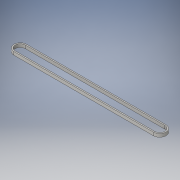
# Autodesk Inventor part: LiftLineWire
Saved by Autodesk Inventor 2016 (Build 200138000, 138)
## iProperties
Created: 2016-12-21
Part Number: LiftLineWire
Material: Generic
Document SubType Name: Modeling
Designer: RoboticsUser
Density: 1 g/cm^3
Appearance: Default
Author: RoboticsUser
Autodesk Inventor part; units mm, degrees
ref_plane "YZ Plane" through (0, 0, 0) normal (1, 0, 0) x (0, 1, 0)
ref_plane "XZ Plane" through (0, 0, 0) normal (0, 1, 0) x (-1, 0, 0)
ref_plane "XY Plane" through (0, 0, 0) normal (0, 0, 1) x (1, 0, 0)
sketch "Sketch1" plane through (0, 0, 0) normal (0, 1, 0) x (-1, 0, 0)
  line L0 (0, 0) -> (304.8083, 0)
  line L1 (304.8083, 0) -> (304.8083, -25.4)
  line L2 (304.8083, -25.4) -> (0, -25.4)
  line L3 (0, -25.4) -> (0, 0)
  dimension "d0" = 25.4
  constraints: 8 end point, 2 parallel, 1 horizontal, 1 perpendicular
  measures "d0" distance of L0.end L1.end
extrude "Extrusion1" add sketch "Sketch1" along normal blind 6.35
fillet "Fillet1" radius 12.7 1 edges at (-304.8083, 3.175, -25.4)
fillet "Fillet2" radius 12.7 1 edges at (-304.8083, 3.175, 0)
fillet "Fillet3" radius 12.7 1 edges at (0, 3.175, 0)
fillet "Fillet4" radius 12.7 1 edges at (0, 3.175, -25.4)
shell "Shell1" thickness 2.54 removed faces 2 at (-198.9723, 6.35, -8.4667) at (-198.9723, 0, -8.4667)
body "Solid1"
